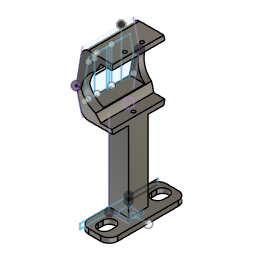
vacuum_gripper v10 (Autodesk Fusion 360 design; units mm, degrees)
Autodesk Fusion 360 part; units mm, degrees
sketch "side1" plane through (0, 0, 0) normal (0, 1, 0) x (1, 0, 0)
  line L0 (-19.73, -38.25) -> (19.73, -38.25)
  circle A0 centre (0, 0) radius 16
  arc A1 (9.6272, -12.7795) -> (4, -21) centre (17.1196, -23.9446) ccw
  arc A2 (-4, -21) -> (-9.6272, -12.7795) centre (-17.1196, -23.9446) ccw
  line L1 (0, 23.75) -> (14, 23.75)
  line L2 (19.73, -38.25) -> (19.73, 23.75)
  line L3 (15.73, 23.75) -> (15.73, -38.25)
  arc A3 (4, 21) -> (9.6272, 12.7795) centre (17.1196, 23.9446) ccw
  arc A4 (-9.6272, 12.7795) -> (-4, 21) centre (-17.1196, 23.9446) ccw
  line L4 (4, 21) -> (-4, 21)
  line L5 (0, -21) -> (4, -21)
  line L6 (0, -21) -> (-4, -21)
  line L7 (4, -21) -> (4, -25)
  line L8 (4, -25) -> (-31, -25)
  line L9 (4, -21) -> (-31, -21)
  line L10 (0, 0) -> (-51, 0)
  line L11 (-31, -21) -> (-43.1244, 0)
  line L12 (-31, -21) -> (-6.7513, -21) construction
  line L13 (-46.5885, -2) -> (-33.3094, -25)
  line L14 (-46.5885, -2) -> (-73.1466, -2) construction
  line L15 (-33.3094, -25) -> (-31, -25)
  line L16 (-46.5885, -2) -> (-47.7432, 0)
  line L17 (4, 21) -> (4, 25)
  line L18 (4, 25) -> (-31, 25)
  line L19 (-33.3094, 25) -> (-31, 25)
  line L20 (-46.5885, 2) -> (-33.3094, 25)
  line L21 (-46.5885, 2) -> (-47.7432, 0)
  line L22 (-31, 21) -> (-43.1244, 0)
  line L23 (4, 21) -> (-31, 21)
  line L24 (-4, 21) -> (-4, 25)
  line L25 (-4, -21) -> (-4, -25)
  circle A5 centre (0, 0) radius 17
  line L26 (-17, 0) -> (-17, -25)
  line L27 (-17, 0) -> (-17, 25)
  line L28 (-17, -25) -> (-21, -25)
  line L29 (-21, -25) -> (-21, 25)
  arc A6 (-9.6272, 12.7795) -> (-4, 25) centre (-36.0311, 32.3437) ccw
  arc A7 (-4, -25) -> (-9.6272, -12.7795) centre (-36.0311, -32.3437) ccw
  dimension "d1" = 19.73
  dimension "d2" = 14
  dimension "d3" = 32
  dimension "d5" = 4
  dimension "d6" = 35
  dimension "d8" = 4
  dimension "d9" = 120
  dimension "d109" = 34
  dimension "d110" = 4
  constraint coincident L3.end L0
  constraint perpendicular L0 L3
  constraint coincident A2.end A0
  constraint parallel L5 L6
  constraint perpendicular L5 L7
  constraint perpendicular L7 L9
  constraint coincident A0.centre L10.start
  constraint horizontal L10
  constraint horizontal L12
  constraint coincident L10 L11.end
  constraint horizontal L14
  constraint parallel L8 L15
  constraint coincident L10 L16.end
  constraint symmetric A1.end L10 A3.start
  constraint symmetric L7.end L10 L17.end
  constraint symmetric L8.end L10 L18.end
  constraint symmetric L9.end L10 L22.start
  constraint symmetric L10 L11.end L22.end
  constraint symmetric L10 L13.start L20.start
  constraint symmetric L10 L13.end L19.start
  constraint symmetric L10 L16.end L21.end
  constraint coincident L18 L24.end
  constraint perpendicular L18 L24
  constraint perpendicular L6 L25
  constraint concentric A0 A5
  constraint coincident A5 L26.start
  constraint coincident L10 L26.start
  constraint coincident L8 L26.end
  constraint perpendicular L8 L26
  constraint coincident L18 L27.end
  constraint perpendicular L18 L27
  constraint coincident L18 L29.end
  constraint perpendicular L18 L29
  constraint symmetric A4.start L10 A2.end
  constraint symmetric L10 L24.end L25.end
  constraint symmetric L10 A6 A7
  measures "d1" distance of L1.start L2.end
  measures "d2" distance of L1.start L1.end
  measures "d3" diameter of A0
  measures "d5" distance of A1.end L7.end
  measures "d6" distance of L7.end L8.end
  measures "d8" distance of L11.end L13.start
  measures "d9" angle of L13 L14
  measures "d109" diameter of A5
  measures "d110" distance of L26.end L28.end
extrude "Extrude1" add sketch "side1" against normal blind 32 contours L4 L17 L18 L23 L24 | L5 L6 L7 L8 L9 L25 | L23 L24 A6 | L23 A5 L27 A6 | L9 L25 A7 | L9 A5 L26 A7 | L18 L23 L27 A6 | L9 L10 L26 L29 | L10 L23 L27 L29 | L8 L9 L26 A7 | L18 L23 L27 L29 | L8 L9 L26 L28 L29
sketch "Sketch15" plane through (-21, 0, 0) normal (-1, 0, 0) x (0, -1, 0)
  line L0 (0, 25) -> (0, -25)
  line L1 (0, -25) -> (32, -25)
  line L2 (32, -25) -> (32, 25)
  line L3 (32, 25) -> (0, 25)
  line L4 (0, 25) -> (-5, 25)
  line L5 (0, 0) -> (-10, 0)
  line L6 (-10, 0) -> (-5, 25)
  line L7 (0, -25) -> (-5, -25)
  line L8 (-10, 0) -> (-5, -25)
  line L9 (32, 0) -> (42, 0)
  line L10 (32, 25) -> (37, 25)
  line L11 (37, 25) -> (42, 0)
  line L12 (32, -25) -> (37, -25)
  line L13 (37, -25) -> (42, 0)
  dimension "d131" = 10
  dimension "d132" = 5
  constraint coincident L0.start L3.end
  constraint perpendicular L0 L4
  constraint coincident L5.start origin
  constraint perpendicular L0 L5
  constraint symmetric L0.start L5 L0.end
  constraint symmetric L4.end L5 L7.end
  constraint symmetric L6.start L5 L8.start
  constraint midpoint L2 L9.start
  constraint perpendicular L2 L9
  constraint coincident L2.end L3.start
  constraint perpendicular L2 L10
  constraint symmetric L11.end L9 L13.end
  constraint symmetric L9 L2.end L1.end
  constraint symmetric L9 L10.end L12.end
  measures "d131" distance of L9.start L9.end
  measures "d132" distance of L2.end L10.end
extrude "Extrude25" add sketch "Sketch15" against normal blind 25 contours L0 L4 L5 L6 | L0 L5 L7 L8 | L2 L9 L10 L11 | L2 L9 L12 L13
sketch "low" plane through (0, 0, -25) normal (0, 0, -1) x (1, 0, 0)
  line L0 (4, -5) -> (4, 37)
  line L1 (33.3094, 49) -> (-4, 49)
  line L2 (4, -5) -> (4, 27)
  line L3 (4, 27) -> (4, 37)
  line L4 (4, -5) -> (-6.3208, -5)
  line L5 (-6.3208, -5) -> (-6.3208, 32)
  line L6 (4, 27) -> (0, 27)
  circle A0 centre (0, 27) radius 1.45
  line L7 (4, 27) -> (-16, 27)
  line L8 (-16, 27) -> (-16, 12)
  line L9 (-16, 27) -> (-16, 52)
  line L10 (0, 27) -> (0, 40)
  line L11 (0, 40) -> (-6.3208, 40)
  line L12 (-6.3208, 40) -> (4, 40)
  line L13 (4, 40) -> (4, 8)
  line L14 (4, 8) -> (-6.3208, 8)
  line L15 (-6.3208, 8) -> (-6.3208, 40)
  line L16 (4, 8) -> (-12, 8)
  line L17 (-12, 8) -> (-12, 24)
  line L18 (-12, 24) -> (4, 24)
  line L19 (4, 24) -> (4, 8)
  line L20 (4, 8) -> (4, 11.4929)
  line L21 (4, 8) -> (4, 11.4929)
  line L22 (4, 37) -> (4, 27)
  line L23 (4, 8) -> (4, 11.4929)
  line L24 (0.3263, 27.9942) -> (-47.4167, 27.9942)
  line L25 (-47.4167, 27.9942) -> (-47.4167, 3.9942)
  line L26 (-47.4167, 3.9942) -> (4, 11.4929)
  line L27 (-47.4167, 3.9942) -> (-44.5304, -15.7964)
  line L28 (-6.3208, -5) -> (-44.5304, -15.7964)
  line L29 (-21, 37) -> (-21, -5)
  line L30 (4, -5) -> (4, 11)
  line L31 (4, 37) -> (-21, 37)
  line L32 (-21, -5) -> (4, -5)
  dimension "d44" = 32
  dimension "d45" = 2.9
  dimension "d46" = 20
  dimension "d49" = 16
  dimension "d50" = 16
  dimension "d68" = 47.743
  dimension "d69" = 24
  dimension "d70" = 20
  dimension "d111" = 16
  constraint coincident L0.start L2.start
  constraint coincident L0.end L3.end
  constraint perpendicular L0 L4
  constraint perpendicular L0 L6
  constraint coincident L6.end A0.centre
  constraint perpendicular L0 L7
  constraint perpendicular L7 L8
  constraint perpendicular L7 L10
  constraint coincident L5 L11.end
  constraint perpendicular L5 L11
  constraint horizontal L12
  constraint vertical L13
  constraint horizontal L14
  constraint vertical L15
  constraint coincident L2 L13.end
  constraint horizontal L16
  constraint vertical L17
  constraint horizontal L18
  constraint vertical L19
  constraint coincident L2 L20.end
  constraint perpendicular L9 L24
  constraint perpendicular L26 L27
  constraint perpendicular L4 L30
  measures "d44" distance of L0.start L2.end
  measures "d45" diameter of A0
  measures "d46" distance of L2.end L7.end
  measures "d49" distance of L13.end L16.end
  measures "d50" distance of L13.end L18.end
  measures "d68" distance of L24.start L24.end
  measures "d69" distance of L24.end L25.end
  measures "d70" distance of L25.end L27.end
  measures "d111" distance of L0.start L30.end
sketch "high" plane through (0, 0, 25) normal (0, 0, 1) x (-1, 0, 0)
  line L0 (-4, 37) -> (-4, -5)
  line L1 (-4, -5) -> (0, 0)
  line L2 (0, 0) -> (4.0005, 0)
  line L3 (4.0005, 0) -> (3.9981, 31.9993)
  line L4 (-4, 37) -> (-4, -5)
  line L5 (4.0005, 0) -> (4.0004, 9)
  line L6 (-4, 37) -> (-4, 26)
  line L7 (1.2978, 2.9621) -> (1.2978, 36)
  line L8 (1.2978, 2.9621) -> (-23.69, 22.9523)
  line L9 (0, 0) -> (47.743, 0)
  line L10 (47.743, 0) -> (47.7359, 32.0026)
  line L11 (47.7359, 32.0026) -> (3.9981, 31.9993)
  line L12 (47.7359, 32.0026) -> (47.7377, 8.0026)
  line L13 (8.9985, 39.354) -> (28.2941, 39.3554)
  line L14 (28.2941, 39.3554) -> (28.2956, 18.1215)
  line L15 (28.2956, 18.1215) -> (9.0001, 18.1215)
  line L16 (8.9985, 39.354) -> (9.0001, 18.1215)
  line L17 (-4, 37) -> (-4, 5)
  line L18 (-4, 5) -> (47.7402, 12.4683)
  line L19 (-0.0011, 32) -> (-0.0009, 23)
  line L20 (-0.0009, 23) -> (0.0002, 9)
  circle A0 centre (-0.0009, 23) radius 1.45
  circle A1 centre (0.0002, 9) radius 1.45
  line L21 (21, -5) -> (21, 37)
  line L22 (21, 37) -> (-4, 37)
  line L23 (-4, -5) -> (21, -5)
  point P0 (0, 49)
  dimension "d17" = 49
  dimension "d18" = 9
  dimension "d40" = 32
  dimension "d64" = 47.743
  dimension "d65" = 24
  dimension "d102" = 32
  dimension "d105" = 9
  dimension "d106" = 14
  dimension "d107" = 2.9
  dimension "d108" = 2.9
  constraint coincident L0.end L1.start
  constraint coincident L1.end L2.start
  constraint coincident L0.start L4.start
  constraint perpendicular L2 L5
  constraint vertical L7
  constraint perpendicular L1 L8
  constraint perpendicular L3 L11
  constraint perpendicular L11 L12
  constraint parallel L11 L13
  constraint perpendicular L13 L14
  constraint perpendicular L13 L16
  constraint parallel L4 L17
  constraint coincident L10 L18.end
  constraint perpendicular L11 L20
  constraint coincident L19.end L20.start
  constraint coincident L20.end A1.centre
  measures "d17" distance of L1.end P0
  measures "d18" distance of L2.end L5.end
  measures "d40" distance of L7.start L8.end
  measures "d64" distance of L1.end L9.end
  measures "d65" distance of L10.end L12.end
  measures "d102" distance of L0.start L17.end
  measures "d105" distance of L19.start L19.end
  measures "d106" distance of L19.end L20.end
  measures "d107" diameter of A0
  measures "d108" diameter of A1
extrude "Extrude4" add sketch "low" along normal blind 70 contours L0 L2 L5 L13 L14 L15 L16 L19 L20 L21 L23 L26 L30 | L5 L15 L16 L17 L26 | L0 L2 L5 L13 L15 L18 L19 L26 | L5 L15 L17 L18 L26
sketch "Sketch6" plane through (0, 0, -95) normal (0, 0, -1) x (1, 0, 0)
  line L0 (-12, 24) -> (-12, 8)
  line L1 (-12, 8) -> (4, 8)
  line L2 (4, 8) -> (4, 24)
  line L3 (-9, 21) -> (-9, 11)
  line L4 (-9, 11) -> (1, 11)
  line L5 (1, 11) -> (1, 21)
  line L6 (1, 21) -> (-9, 21)
  circle A0 centre (-9, 21) radius 1.45
  circle A1 centre (-9, 11) radius 1.45
  circle A2 centre (1, 21) radius 1.45
  circle A3 centre (1, 11) radius 1.45
  circle A4 centre (0, 16) radius 3.1
  line L7 (0, 16) -> (12, 16)
  line L8 (4, 24) -> (-12, 24)
  circle A5 centre (0, 16) radius 1.45
  dimension "d51" = 2.9
  dimension "d52" = 2.9
  dimension "d53" = 2.9
  dimension "d54" = 2.9
  dimension "d55" = 6.2
  dimension "d88" = 12
  dimension "d118" = 2.9
  constraint perpendicular L3 L4
  constraint perpendicular L4 L5
  constraint perpendicular L3 L6
  constraint coincident L3.start L6.end
  constraint coincident L3.end L4.start
  constraint coincident L5.end L6.start
  constraint coincident L4.end L5.start
  constraint coincident A4.centre L7.start
  constraint perpendicular L2 L7
  constraint concentric A4 A5
  measures "d51" diameter of A0
  measures "d52" diameter of A1
  measures "d53" diameter of A2
  measures "d54" diameter of A3
  measures "d55" diameter of A4
  measures "d88" distance of A4.centre L7.end
  measures "d118" diameter of A5
sketch "Sketch8" plane through (-12, 0, 0) normal (-1, 0, 0) x (0, -1, 0)
  line L0 (24, -25) -> (8, -25)
  line L1 (8, -25) -> (8, -95)
  line L2 (8, -95) -> (24, -95)
  line L3 (8, -95) -> (-16, -95)
  line L4 (24, -95) -> (48, -95)
  line L5 (-16, -95) -> (-16, -91)
  line L6 (-16, -91) -> (8, -91)
  line L7 (48, -95) -> (48, -91)
  line L8 (48, -91) -> (24, -91)
  line L9 (8, -91) -> (24, -91)
  line L10 (24, -95) -> (24, -25)
  dimension "d84" = 4
  dimension "d85" = 4
  constraint coincident L1.end L2.start
  constraint perpendicular L1 L3
  constraint coincident L2.end L4.start
  constraint perpendicular L3 L5
  constraint coincident L1 L6.end
  constraint perpendicular L1 L6
  constraint perpendicular L4 L7
  measures "d84" distance of L3.end L5.end
  measures "d85" distance of L4.end L7.end
extrude "Extrude14" add sketch "Sketch8" against normal blind 16 contours L4 L7 L8 L10 | L1 L3 L5 L6
extrude "Extrude15" add sketch "Sketch8" against normal blind 24 contours L4 L7 L8 L10 | L1 L3 L5 L6
extrude "Extrude16" add sketch "Sketch8" against normal blind 8 from surface at -16 contours L1 L2 L9 L10
fillet "Fillet1" radius 7 4 edges at (12, -48, -93) (-12, -48, -93) (12, 16, -93) (-12, 16, -93)
sketch "Sketch10" plane through (0, -8, 0) normal (0, 1, 0) x (-1, 0, 0)
  line L0 (-4, -91) -> (12, -91)
  line L1 (12, -91) -> (12, -25)
  line L2 (-4, -25) -> (-4, -91)
  arc A0 through (59.7468, -47.5288, -7.4579) (51.3094, -30.3246, -7.1548) (38.4266, -16.1367, -7.1025)
  line L3 (12, -25) -> (-4, -25)
sketch "Sketch13" plane through (-21, 0, 0) normal (-1, 0, 0) x (0, -1, 0)
  line L0 (-5, -25) -> (37, -25)
  line L1 (37, 25) -> (-5, 25)
  line L2 (5, 25) -> (5, 15)
  line L3 (32, 12) -> (27, 12)
  line L4 (5, 15) -> (27, 15)
  line L5 (5, 15) -> (27, 15)
  line L6 (27, 15) -> (27, -14.6713)
  line L7 (27, -14.6713) -> (5, -14.6713)
  line L8 (5, -14.6713) -> (5, 15)
  line L9 (37, -25) -> (42, 0)
  line L10 (42, 0) -> (37, 25)
  line L11 (-5, 25) -> (-10, 0)
  line L12 (-10, 0) -> (-5, -25)
  line L13 (5, 15) -> (-2, 15)
  line L14 (27, 0) -> (5, 0)
  line L15 (5, 0) -> (-10, 0)
  line L16 (-10, 0) -> (-5, 0)
  line L17 (-2, 15) -> (-5, 0)
  line L18 (5, -14.6713) -> (-5, -14.6713)
  line L19 (-5, 0) -> (-2, -14.6713)
  line L20 (15, 15) -> (15, -14.6713)
  line L21 (25, 15) -> (32, 15)
  line L22 (32, 15) -> (35, 0)
  line L23 (35, 0) -> (32, -14.6713)
  line L24 (25, -14.6713) -> (35, -14.6713)
  line L25 (15, 15) -> (17, 15)
  line L26 (17, -14.6713) -> (15, -14.6713)
  line L27 (17, 15) -> (17, -14.6713)
  line L28 (13, 15) -> (13, -14.6713)
  dimension "d140" = 5
  constraint coincident L1 L2.start
  constraint perpendicular L2 L4
  constraint horizontal L5
  constraint vertical L6
  constraint horizontal L7
  constraint vertical L8
  constraint perpendicular L8 L13
  constraint coincident L6 L14.start
  constraint coincident L8 L14.end
  constraint perpendicular L8 L14
  constraint coincident L11.end L12.start
  constraint parallel L14 L15
  constraint parallel L15 L16
  constraint perpendicular L8 L18
  constraint coincident L18 L19.end
  constraint coincident L4 L20.start
  constraint coincident L7 L20.end
  constraint perpendicular L7 L20
  constraint symmetric L2.end L20 L21.start
  constraint symmetric L7.end L20 L24.start
  constraint symmetric L13.end L20 L21.end
  constraint symmetric L16.end L20 L22.end
  constraint symmetric L18.end L20 L24.end
  constraint symmetric L19.end L20 L23.end
  constraint coincident L5 L25.end
  constraint perpendicular L20 L25
  constraint coincident L7 L26.start
  constraint perpendicular L26 L27
  constraint symmetric L20 L25.end L28.start
  constraint symmetric L20 L26.start L28.end
  measures "d140" distance of L11.end L16.end
extrude "Extrude21" cut sketch "high" against normal blind 4 contours L7 A1 | L7 A1 | L7 L19 L20 A0 | L7 A0 | L19 L20 A0
extrude "Extrude22" cut sketch "Sketch6" against normal blind 72.3 contours L5 A4 L7 A5 | L5 A4 A5 | L5 L7 A5 | L5 A5 | L5 A4 L7 A5 | L5 L7 A5
extrude "Extrude23" cut sketch "Sketch6" against normal blind 76 contours L5 L7 A5 | L5 A5 | L5 L7 A5
sketch "Sketch14" plane through (0, 0, -95) normal (0, 0, -1) x (1, 0, 0)
  circle A0 centre (0, 16) radius 3.1
  arc A1 (-12, -9) -> (-5, -16) centre (-5, -9) ccw
  line L0 (-5, -16) -> (5, -16)
  arc A2 (5, -16) -> (12, -9) centre (5, -9) ccw
  line L1 (12, -9) -> (12, 41)
  arc A3 (12, 41) -> (5, 48) centre (5, 41) ccw
  line L2 (5, 48) -> (-5, 48)
  arc A4 (-5, 48) -> (-12, 41) centre (-5, 41) ccw
  line L3 (-12, 41) -> (-12, -9)
  line L4 (0, 48) -> (0, 40)
  line L5 (0, -16) -> (0, -8)
  line L6 (0, 40) -> (5.1, 40)
  line L7 (0, 40) -> (-5.1, 40)
  circle A5 centre (0, 40) radius 5.1
  line L8 (-5.1, 40) -> (-5.1, 36)
  line L9 (-5.1, 36) -> (5.1, 36)
  line L10 (5.1, 36) -> (5.1, 40)
  circle A6 centre (0, 36) radius 5.1
  line L11 (0, 16) -> (12, 16)
  line L12 (0, 16) -> (12, 16)
  circle A7 centre (0, -8) radius 5.1
  line L13 (5.1, -4) -> (5.1, -8)
  circle A8 centre (0, -4) radius 5.1
  line L14 (-5.1, -8) -> (-5.1, -4)
  dimension "d121" = 8
  dimension "d122" = 8
  dimension "d123" = 5.1
  dimension "d124" = 5.1
  dimension "d125" = 10.2
  dimension "d126" = 10.2
  constraint midpoint L2 L4.start
  constraint perpendicular L2 L4
  constraint midpoint L0 L5.start
  constraint perpendicular L0 L5
  constraint perpendicular L4 L6
  constraint perpendicular L4 L7
  constraint coincident L4.end L6.start
  constraint tangent A5 L8
  constraint perpendicular L7 L8
  constraint perpendicular L8 L9
  constraint tangent A5 L10
  constraint midpoint L9 A6.centre
  constraint coincident A0.centre L11.start
  constraint midpoint L1 L11.end
  constraint symmetric L6.end L12 L13.end
  constraint symmetric L7.end L12 L14.start
  constraint symmetric A5 L12 A7
  constraint symmetric L8.end L12 L14.end
  constraint symmetric L9.end L12 L13.start
  constraint symmetric A6 L12 A8
  measures "d121" distance of L4.start L4.end
  measures "d122" distance of L5.start L5.end
  measures "d123" distance of L4.end L6.end
  measures "d124" distance of L4.end L7.end
  measures "d125" diameter of A5
  measures "d126" diameter of A6
extrude "Extrude24" cut sketch "Sketch14" against normal blind 4 contours L4 L6 A5 A6 | L4 L7 A5 A6 | L4 L6 A6 | L4 L7 A6 | L6 A5 A6 | A5 L10 A6 | L7 A5 A6 | A5 L8 A6 | L6 L7 A5 L9 A6 | A5 L9 A6 | A5 L9 A6 | A5 L9 A6 | A5 L9 | L5 A7 A8 | L5 A7 A8 | A7 A8 | A7 A8 L14 | A7 L13 A8 | A7 A8
extrude "Extrude26" cut 1 faces at (-0.0596, -32, 4.9678) along direction (0, -1, 0) blind 13
extrude "Extrude27" cut 1 faces at (-0.0596, 0, 4.9678) along direction (0, 1, 0) blind 16
sketch "Sketch16" plane through (-21, 0, 0) normal (-1, 0, 0) x (0, -1, 0)
  line L0 (-5, -25) -> (37, -25)
  line L1 (37, -25) -> (42, 0)
  line L2 (42, 0) -> (37, 25)
  line L3 (37, 25) -> (-5, 25)
  line L4 (-5, 25) -> (-10, 0)
  line L5 (-10, 0) -> (-5, -25)
extrude "Extrude28" cut sketch "Sketch13" against normal blind 25 contours L8 L13 L15 L17 | L8 L15 L18 L19 | L7 L8 L14 L28 | L4 L5 L8 L14 L28 | L4 L5 L14 L20 L28 | L7 L14 L20 L28 | L4 L5 L14 L20 L25 L27 | L7 L14 L20 L26 L27 | L4 L5 L6 L14 L21 L27 | L6 L7 L14 L24 L27 | L6 L21 L22 L23 L24
fillet "Fillet3" radius 5 2 edges at (-21, -16, 25) (-21, -16, -25)
